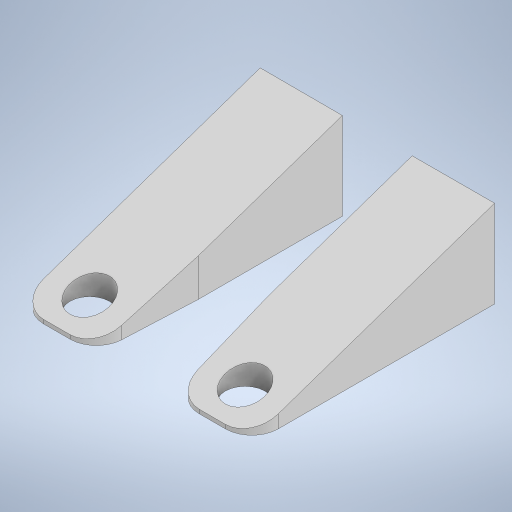
# Autodesk Inventor part: 20degree spacer
Saved by Autodesk Inventor 2023.2 (Build 272271030, 271C)
## iProperties
Created: 2023-04-24
Part Number: 20degree spacer
Material: Generic
Document SubType Name: Modeling
Designer: daanj
Density: 1 g/cm^3
Appearance: Default
Author: daanj
Autodesk Inventor part; units mm, degrees
ref_plane "YZ Plane" through (0, 0, 0) normal (1, 0, 0) x (0, 1, 0)
ref_plane "XZ Plane" through (0, 0, 0) normal (0, 1, 0) x (-1, 0, 0)
ref_plane "XY Plane" through (0, 0, 0) normal (0, 0, 1) x (1, 0, 0)
sketch "Sketch1" plane through (0, 0, 0) normal (0, 1, 0) x (-1, 0, 0)
  line L0 (-8.9015, 1.1073) -> (-8.9015, 17.5545)
  line L1 (-2.6515, 1.1073) -> (-8.9015, 1.1073)
  line L2 (-2.6515, 12.0754) -> (-2.6515, 1.1172)
  line L3 (-2.9035, 17.6442) -> (-2.6515, 12.0754)
  ellipse E0 centre (-4.9015, 17.5545) end of major axis (-2.9015, 17.5545) minor radius 1.9924 (-2.9035, 17.6442) -> (-4.9015, 19.5469) ccw
  line L4 (-6.9015, 19.5469) -> (-4.9015, 19.5469)
  ellipse E1 centre (-6.9015, 17.5545) end of major axis (-8.9015, 17.5545) minor radius 1.9924 (-6.9015, 19.5469) -> (-8.9015, 17.5545) ccw
  ellipse E2 centre (-5.9015, 17.0564) end of major axis (-4.4015, 17.0564) minor radius 1.4943
  line L5 (-8.9015, 1.1073) -> (-8.9015, 1.3688)
  line L6 (-8.9015, 1.1073) -> (-2.6515, 1.1172)
  line L7 (-2.6515, 1.1172) -> (-2.6515, 12.0754)
  line L8 (-2.6515, 12.0754) -> (-2.9035, 17.6442)
  line L9 (-8.9015, 1.1073) -> (-8.9015, 17.5545)
  line L10 (-6.9015, 19.5469) -> (-4.9015, 19.5469)
  circle A0 centre (-5.9015, 17.0564) radius 1.5
  line L11 (8.9015, 1.1073) -> (8.9015, 17.5545)
  line L12 (2.6515, 1.1073) -> (8.9015, 1.1073)
  line L13 (2.6515, 12.0754) -> (2.6515, 1.1172)
  line L14 (2.9035, 17.6442) -> (2.6515, 12.0754)
  ellipse E3 centre (4.9015, 17.5545) end of major axis (2.9015, 17.5545) minor radius 1.9924 (4.9015, 19.5469) -> (2.9035, 17.6442) ccw
  line L15 (6.9015, 19.5469) -> (4.9015, 19.5469)
  ellipse E4 centre (6.9015, 17.5545) end of major axis (8.9015, 17.5545) minor radius 1.9924 (8.9015, 17.5545) -> (6.9015, 19.5469) ccw
  ellipse E5 centre (5.9015, 17.0564) end of major axis (4.4015, 17.0564) minor radius 1.4943
  line L16 (8.9015, 1.1073) -> (8.9015, 1.3688)
  line L17 (8.9015, 1.1073) -> (2.6515, 1.1172)
  line L18 (2.6515, 1.1172) -> (2.6515, 12.0754)
  line L19 (2.6515, 12.0754) -> (2.9035, 17.6442)
  line L20 (8.9015, 1.1073) -> (8.9015, 17.5545)
  line L21 (6.9015, 19.5469) -> (4.9015, 19.5469)
  circle A1 centre (5.9015, 17.0564) radius 1.5
  point P0 (0, 0)
  point P1 (-18.0813, 13.3212)
  constraints: 44 end point, 3 centre point, 2 coincident, 2 collinear, 2 point on line, 1 concentric, 1 horizontal, 1 vertical, 18 other
extrude "Extrusion1" add sketch "Sketch1" along normal blind 10
sketch "Sketch2" plane through (8.9015, 0, 17.5545) normal (1, 0, 0) x (0, 0, -1)
  line L0 (16.4472, 6.631) -> (-1.9924, 0.3)
  line L1 (16.4472, 6.631) -> (16.4472, 13.2162)
  line L2 (16.4472, 13.2162) -> (-1.9924, 13.2162)
  line L3 (-1.9924, 13.2162) -> (-1.9924, 0.3)
  line L4 (0, 0) -> (-1.9924, 0) projected
  point P0 (17.5545, 0)
  point P1 (16.4472, 0)
  dimension "d5" = 6.631
  dimension "d8" = 0.3
  constraints: 8 end point, 2 perpendicular, 1 vertical
  measures "d5" distance of L0.start point (16.447, 0)
  measures "d8" distance from line of L0.end L4
extrude "Extrusion2" cut sketch "Sketch2" against normal through all
body "Solid1"
